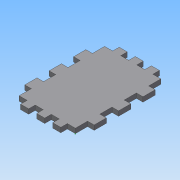
# Autodesk Inventor part: Level
Saved by Autodesk Inventor 2015 (Build 190159000, 159)
## iProperties
Created: 2014-11-11
Part Number: Level
Material: Generic
Document SubType Name: Modeling
Designer: 0
Density: 1 g/cm^3
Appearance: Default
BaseWidth: 4.560 in
BaseLength: 3.000 in
Thickness: 0.250 in
WallConSpace: 0.651 in
WallConA: 0.350 in
WallConB: 0.651 in
PerpSpace: 0.429 in
PerpB: 0.429 in
PerpA: 0.350 in
Author: 0
Autodesk Inventor part; units mm, degrees
ref_plane "YZ Plane" through (0, 0, 0) normal (1, 0, 0) x (0, 1, 0)
ref_plane "XZ Plane" through (0, 0, 0) normal (0, 1, 0) x (-1, 0, 0)
ref_plane "XY Plane" through (0, 0, 0) normal (0, 0, 1) x (1, 0, 0)
sketch "Sketch1" plane through (0, 0, 0) normal (0, 1, 0) x (-1, 0, 0)
  point P0 (0, 0)
sketch "Sketch2" plane through (0, 0, 0) normal (0, 1, 0) x (-1, 0, 0)
  line L0 (0, 0) -> (76.2, 0)
  line L1 (76.2, 0) -> (76.2, -115.824)
  line L2 (76.2, -115.824) -> (0, -115.824)
  line L3 (0, -115.824) -> (0, 0)
  dimension "BaseLength" = 76.2
  dimension "BaseWidth" = 115.824
  constraints: 8 end point, 2 parallel, 1 horizontal, 1 perpendicular
  measures "BaseLength" distance of L1.end L2.end
  measures "BaseWidth" distance of L0.end L1.end
extrude "Base Extrusion" add sketch "Sketch2" along normal blind 6.35
sketch "Sketch3" plane through (0, 0, 0) normal (0, 1, 0) x (-1, 0, 0)
  line L0 (76.2, 0) -> (0, 0) projected
  line L1 (0, 0) -> (0, -115.824) projected
  line L2 (0, -115.824) -> (76.2, -115.824) projected
  line L3 (76.2, -115.824) -> (76.2, 0) projected
  line L4 (10.8857, 0) -> (21.7714, 0)
  line L5 (21.7714, 0) -> (21.7714, 8.89)
  line L6 (21.7714, 8.89) -> (10.8857, 8.89)
  line L7 (10.8857, 8.89) -> (10.8857, 0)
  line L8 (32.6571, 0) -> (43.5429, 0)
  line L9 (43.5429, 0) -> (43.5429, 8.89)
  line L10 (43.5429, 8.89) -> (32.6571, 8.89)
  line L11 (32.6571, 8.89) -> (32.6571, 0)
  line L12 (54.4286, 0) -> (65.3143, 0)
  line L13 (65.3143, 0) -> (65.3143, 8.89)
  line L14 (65.3143, 8.89) -> (54.4286, 8.89)
  line L15 (54.4286, 8.89) -> (54.4286, 0)
  line L16 (76.2, -57.912) -> (0, -57.912) construction
  line L17 (76.2, -115.824) -> (0, -115.824)
  line L18 (10.8857, -115.824) -> (21.7714, -115.824)
  line L19 (21.7714, -115.824) -> (21.7714, -124.714)
  line L20 (21.7714, -124.714) -> (10.8857, -124.714)
  line L21 (10.8857, -124.714) -> (10.8857, -115.824)
  line L22 (43.5429, -115.824) -> (43.5429, -124.714)
  line L23 (43.5429, -124.714) -> (32.6571, -124.714)
  line L24 (32.6571, -124.714) -> (32.6571, -115.824)
  line L25 (32.6571, -115.824) -> (43.5429, -115.824)
  line L26 (65.3143, -115.824) -> (65.3143, -124.714)
  line L27 (65.3143, -124.714) -> (54.4286, -124.714)
  line L28 (54.4286, -124.714) -> (54.4286, -115.824)
  line L29 (54.4286, -115.824) -> (65.3143, -115.824)
  line L30 (38.1, 0) -> (38.1, -115.824) construction
  line L31 (0, -16.5463) -> (-8.89, -16.5463)
  line L32 (-8.89, -16.5463) -> (-8.89, -33.0926)
  line L33 (-8.89, -33.0926) -> (0, -33.0926)
  line L34 (0, -33.0926) -> (0, -16.5463)
  line L35 (0, -49.6389) -> (-8.89, -49.6389)
  line L36 (-8.89, -49.6389) -> (-8.89, -66.1851)
  line L37 (-8.89, -66.1851) -> (0, -66.1851)
  line L38 (0, -66.1851) -> (0, -49.6389)
  line L39 (0, -82.7314) -> (-8.89, -82.7314)
  line L40 (-8.89, -82.7314) -> (-8.89, -99.2777)
  line L41 (-8.89, -99.2777) -> (0, -99.2777)
  line L42 (0, -99.2777) -> (0, -82.7314)
  line L43 (76.2, 0) -> (76.2, -115.824)
  line L44 (76.2, -16.5463) -> (85.09, -16.5463)
  line L45 (85.09, -16.5463) -> (85.09, -33.0926)
  line L46 (85.09, -33.0926) -> (76.2, -33.0926)
  line L47 (76.2, -33.0926) -> (76.2, -16.5463)
  line L48 (76.2, -49.6389) -> (85.09, -49.6389)
  line L49 (85.09, -49.6389) -> (85.09, -66.1851)
  line L50 (85.09, -66.1851) -> (76.2, -66.1851)
  line L51 (76.2, -66.1851) -> (76.2, -49.6389)
  line L52 (76.2, -82.7314) -> (85.09, -82.7314)
  line L53 (85.09, -82.7314) -> (85.09, -99.2777)
  line L54 (85.09, -99.2777) -> (76.2, -99.2777)
  line L55 (76.2, -99.2777) -> (76.2, -82.7314)
  dimension "d4" = 10.8857
  dimension "d5" = 8.89
  dimension "PerpSpace" = 10.8857
  dimension "d7" = 10.8857
  dimension "d8" = 8.89
  dimension "PerpB" = 10.8857
  dimension "PerpA" = 8.89
  dimension "d11" = 10.8857
  dimension "d13" = 10.8857
  dimension "d14" = 76.2
  dimension "WallConSpace" = 16.5463
  dimension "d16" = 115.824
  dimension "WallConA" = 8.89
  dimension "WallConB" = 16.5463
  dimension "d19" = 8.89
  dimension "d20" = 16.5463
  dimension "d21" = 8.89
  dimension "d22" = 16.5463
  dimension "d23" = 16.5463
  dimension "d24" = 16.5463
  constraints: 104 end point, 24 symmetric about line, 12 parallel, 6 collinear, 6 horizontal, 6 perpendicular, 4 midpoint
  measures "d4" distance of L6.end L5.end
  measures "d5" distance of L5.end L4.end
  measures "PerpSpace" distance between parallel lines of L1 L7
  measures "d7" distance of L10.end L9.end
  measures "d8" distance of L9.end L9.start
  measures "PerpB" distance of L14.end L13.end
  measures "PerpA" distance of L13.end L13.start
  measures "d11" distance between parallel lines of L5 L11
  measures "d13" distance between parallel lines of L9 L15
  measures "d14" distance of L0.start L0.end
  measures "WallConSpace" distance between parallel lines of L0 L31
  measures "d16" distance of L0.end L1.end
  measures "WallConA" distance of L32.end L33.end
  measures "WallConB" distance of L31.end L32.end
  measures "d19" distance of L35.start L35.end
  measures "d20" distance of L35.end L36.end
  measures "d21" distance of L39.start L39.end
  measures "d22" distance of L39.end L40.end
  measures "d23" distance between parallel lines of L33 L35
  measures "d24" distance between parallel lines of L37 L39
extrude "Connections" add sketch "Sketch3" along normal blind 6.35 contours L0 L15 L14 L13 | L44 L45 L46 L3 | L0 L11 L10 L9 | L48 L49 L50 L3 | L0 L7 L6 L5 | L52 L53 L54 L3 | L1 L33 L32 L31 | L26 L27 L28 L2 | L1 L37 L36 L35 | L22 L23 L24 L2 | L1 L41 L40 L39 | L19 L20 L21 L2
equation "\"d4\" = 0.142857 * d14"
equation "\"PerpSpace\" = -0.75 * d4 + 0.25 * d14"
equation "\"d7\" = d4"
equation "\"d8\" = d5"
equation "\"PerpB\" = d4"
equation "\"PerpA\" = d5"
equation "\"d11\" = PerpSpace"
equation "\"d13\" = PerpSpace"
equation "\"WallConSpace\" = -0.75 * WallConB + 0.25 * d16"
equation "\"WallConB\" = 0.142857 * d16"
equation "\"d19\" = WallConA"
equation "\"d20\" = WallConB"
equation "\"d21\" = WallConA"
equation "\"d22\" = WallConB"
equation "\"d23\" = WallConSpace"
equation "\"d24\" = WallConSpace"
body "Solid1"
